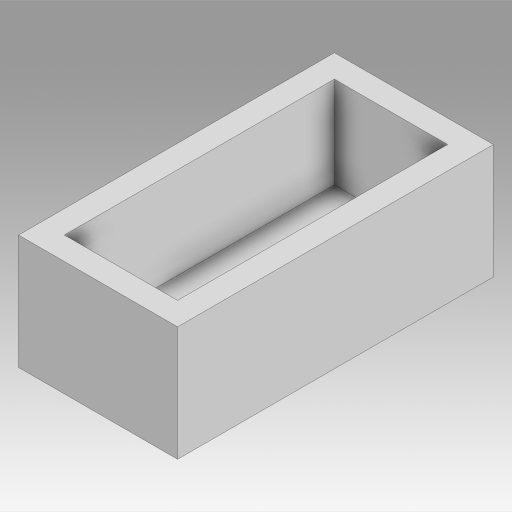
# Autodesk Inventor part: BOX
Saved by Autodesk Inventor 2023 (Build 270158000, 158)
## iProperties
Created: 2025-08-22
Part Number: BOX
Material: Generic
Document SubType Name: Modeling
Designer: NELLY NDUNG'U
Density: 1 g/cm^3
Appearance: Default
Author: NELLY NDUNG'U
Autodesk Inventor part; units mm, degrees
ref_plane "YZ Plane" through (0, 0, 0) normal (1, 0, 0) x (0, 1, 0)
ref_plane "XZ Plane" through (0, 0, 0) normal (0, 1, 0) x (-1, 0, 0)
ref_plane "XY Plane" through (0, 0, 0) normal (0, 0, 1) x (1, 0, 0)
sketch "Sketch1" plane through (0, 0, 0) normal (0, 1, 0) x (-1, 0, 0)
  line L0 (8.8039, 17.4877) -> (-8.8039, 17.4877)
  line L1 (-8.8039, 17.4877) -> (-8.8039, -17.4877)
  line L2 (-8.8039, -17.4877) -> (8.8039, -17.4877)
  line L3 (8.8039, -17.4877) -> (8.8039, 17.4877)
  line L4 (8.8039, 17.4877) -> (-8.8039, -17.4877) construction
  line L5 (-8.8039, 17.4877) -> (8.8039, -17.4877) construction
  point P0 (0, 0)
  constraints: 12 end point, 2 midpoint, 2 parallel, 1 horizontal, 1 perpendicular
extrude "Extrusion1" add sketch "Sketch1" along normal blind 12.7
shell "Shell1" thickness 2.54 removed faces 1 at (2.9346, 12.7, 5.8292)
body "Solid1"
